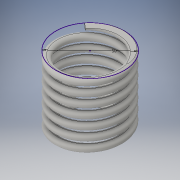
# Autodesk Inventor part: Spring
Saved by Autodesk Inventor 2016 (Build 200138000, 138)
## iProperties
Created: 2015-09-12
Part Number: Spring
Material: Generic
Document SubType Name: Modeling
Designer: nightstalker
Density: 1 g/cm^3
Appearance: Default
Mass: 19406.9 g
Surface Area: 15782.6 cm^2
Volume: 19406.9 cm^3
Author: nightstalker
Autodesk Inventor part; units mm, degrees
ref_plane "YZ Plane" through (0, 0, 0) normal (1, 0, 0) x (0, 1, 0)
ref_plane "XZ Plane" through (0, 0, 0) normal (0, 1, 0) x (-1, 0, 0)
ref_plane "XY Plane" through (0, 0, 0) normal (0, 0, 1) x (1, 0, 0)
sketch "Sketch13" plane through (0, 0, 0) normal (0, 1, 0) x (-1, 0, 0)
  circle A0 centre (0, 0) radius 250
  dimension "d28" = 500
  constraints: 1 centre point, 1 coincident
  measures "d28" diameter of A0
extrude "Extrusion5" add sketch "Sketch13" along normal blind 500
sketch "Sketch14" plane through (0, 0, 0) normal (1, 0, 0) x (0, 1, 0)
  line L0 (0, 250) -> (500, 250) projected
  line L1 (500, 250) -> (500, -250) projected
  line L2 (500, -250) -> (0, -250) projected
  line L3 (0, -250) -> (0, 250) projected
  line L4 (500, 0) -> (0, 0)
  circle A0 centre (0, -225) radius 25
  dimension "d31" = 50
  constraints: 2 end point, 1 centre point, 1 horizontal, 1 midpoint, 1 point on line, 1 tangent
  measures "d31" diameter of A0
coil "Coil3" sketch "Sketch14" operation intersect axis through (0, 500, 0) along (0, 1, 0) pitch 70 turns 7.142857 hand right contours A0 L3 | L3 A0
sketch "Sketch15" plane through (0, 500, 0) normal (0, 1, 0) x (1, 0, 0)
  circle A0 centre (0, 0) radius 250
  dimension "d40" = 500
  constraints: 1 centre point, 1 coincident
  measures "d40" diameter of A0
body "Solid5"
